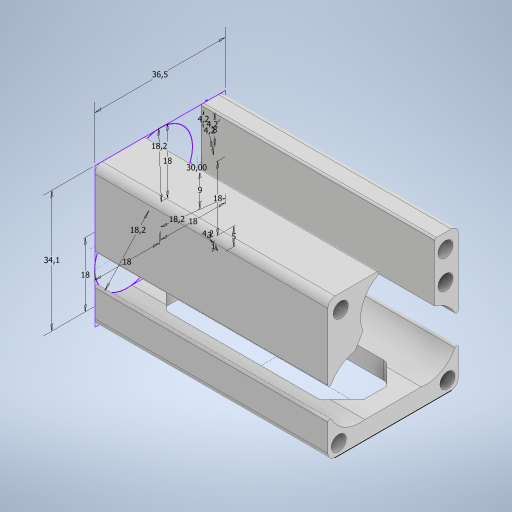
# Autodesk Inventor part: left_akkum
Saved by Autodesk Inventor 2023 (Build 270158000, 158)
## iProperties
Created: 2026-02-15
Part Number: left_akkum
Material: Типовые
Document SubType Name: Modeling
Designer: garin
Density: 1 g/cm^3
Appearance: По умолчанию
Author: garin
Autodesk Inventor part; units mm, degrees
ref_plane "YZ Plane" through (0, 0, 0) normal (1, 0, 0) x (0, 1, 0)
ref_plane "XZ Plane" through (0, 0, 0) normal (0, 1, 0) x (-1, 0, 0)
sketch "Эскиз1" plane through (0, 0, 0) normal (1, 0, 0) x (0, 1, 0)
  line L0 (-16.6, -18.25) -> (17.5, -18.25)
  line L1 (17.5, -18.25) -> (17.5, 18.25)
  line L2 (17.5, 18.25) -> (-16.6, 18.25)
  line L3 (-16.6, 18.25) -> (-16.6, -18.25)
  line L4 (17.5, 0) -> (-0.5, 0) construction
  circle A0 centre (8.5, 0) radius 9
  line L5 (-16.6, -18.25) -> (1.4, -18.25) construction
  line L6 (-7.6, -18.25) -> (-7.6, -0.25) construction
  circle A1 centre (-7.6, -9.25) radius 9
  line L7 (-16.6, 18.25) -> (1.4, 18.25) construction
  line L8 (-7.6, 18.25) -> (-7.6, 0.25) construction
  circle A2 centre (-7.6, 9.25) radius 9
  line L9 (-16.6, -18.25) -> (-16.6, -15.75)
  line L10 (-16.6, 18.25) -> (-21.6, 18.25)
  line L11 (-21.6, 18.25) -> (-21.6, -18.25)
  line L12 (-21.6, -18.25) -> (-16.6, -18.25)
  line L13 (-16.6, -18.25) -> (-16.6, 18.25)
  circle A3 centre (-18.6, -15.2) radius 1.5
  circle A4 centre (-18.6, -15.2) radius 2.1
  line L14 (-21.6, 18.25) -> (17.5, 18.25) construction
  line L15 (-2.05, 18.25) -> (-2.05, -18.25) construction
  circle A5 centre (13.4, -14.65) radius 1.5
  circle A6 centre (13.4, -14.65) radius 2.1
  circle A7 centre (8.5, 0) radius 9.1
  circle A8 centre (-7.6, 9.25) radius 9.1
  circle A9 centre (-7.6, -9.25) radius 9.1
  line L16 (-7.6, -0.15) -> (1.4, -0.15) construction
  line L17 (1.4, -0.15) -> (1.4, -10.5954) construction
  line L18 (1.4, -10.5954) -> (-7.6, -10.5954) construction
  line L19 (-7.6, -10.5954) -> (-7.6, -0.15) construction
  line L20 (1.4, -10.5954) -> (5.1186, -8.4484)
  line L21 (1.4, -10.5954) -> (5.6939, -10.5954) construction
  line L22 (1.4, 10.5954) -> (5.1186, 8.4484)
  line L23 (-16.7, 9.25) -> (-21.6, 9.25)
  line L24 (-16.7, -9.25) -> (-21.6, -9.25)
  line L25 (17.5, -11.65) -> (1.2036, -11.5536)
  line L26 (15.5, -18.25) -> (15.5, -11.6382) construction
  line L27 (11.3933, -16.75) -> (17.6, -16.75) construction
  line L28 (15.5, -16.75) -> (11.3, -16.75) construction
  line L29 (11.3, -16.75) -> (11.3, -12.55) construction
  line L30 (11.3, -12.55) -> (15.5, -12.55) construction
  line L31 (15.5, -12.55) -> (15.5, -16.75) construction
  line L32 (15.5, -14.65) -> (11.3, -14.65) construction
  line L33 (13.4, -12.55) -> (13.4, -16.75) construction
  circle A10 centre (13.4, 14.65) radius 1.5
  circle A11 centre (13.4, 14.65) radius 2.1
  line L34 (13.4, -14.65) -> (-21.6, -14.65) construction
  line L35 (-18.1, -14.65) -> (-19.1, -14.65) construction
  line L36 (-19.1, -15.75) -> (-18.1, -14.65) construction
  circle A12 centre (-18.6, 15.2) radius 1.5
  circle A13 centre (-18.6, 15.2) radius 2.1
  line L37 (13.4, -14.65) -> (5.4, -14.65)
  circle A14 centre (5.4, -14.65) radius 2.1
  point P0 (0, 0)
  point P1 (-8.9454, -18.25)
  point P2 (-8.9454, 18.25)
  point P3 (-6.2546, -18.25)
  point P4 (17.5, -1.3454)
  point P5 (17.5, 1.3454)
  point P6 (-6.2546, 18.25)
  point P7 (0.6455, -13.1)
  point P8 (17.5, -13.1)
  point P9 (-16.6, -7.9046)
  point P10 (-16.6, 7.9046)
  point P11 (-16.6, -10.5954)
  dimension "d13" = 18.2
  dimension "d14" = 18.2
  dimension "d0" = 34.1
  dimension "d1" = 36.5
  dimension "d2" = 18
  dimension "d3" = 18
  dimension "d4" = 18
  dimension "d5" = 18
  dimension "d6" = 18
  dimension "d8" = 5
  dimension "d11" = 3
  dimension "d12" = 4.2
  dimension "d15" = 18.2
  dimension "d16" = 9
  dimension "d17" = 30
  dimension "d27" = 4.2
  dimension "d28" = 4.2
  dimension "d29" = 1
  dimension "d48" = 8
  dimension "d49" = 4.2
  constraints: 76 end point, 18 point on line, 13 midpoint, 10 centre point, 9 coincident, 9 perpendicular, 8 parallel, 6 symmetric about line, 5 horizontal, 5 point on circle, 2 vertical alignment, 1 collinear, 1 equal length, 1 horizontal alignment, 1 vertical, 16 other
  measures "d0" distance of L2.end L1.end
  measures "d1" distance of L1.end L0.end
  measures "d2" distance of L4.start L4.end
  measures "d3" distance of L0.start L5.end
  measures "d4" distance of L6.start L6.end
  measures "d5" distance of L2.end L7.end
  measures "d6" distance of L8.start L8.end
  measures "d8" distance of L12.end L11.end
  measures "d11" diameter of A3
  measures "d12" diameter of A4
  measures "d15" diameter of A9
  measures "d16" distance of L17.end L18.end
  measures "d17" angle of L21 L20
  measures "d27" distance of L29.end L30.end
  measures "d28" distance of L28.end L29.end
  measures "d29" distance of L35.start L35.end
  measures "d48" distance of L34.start L37.end
  measures "d49" diameter of A14
extrude "Выдавливание3" add sketch "Эскиз1" along normal blind 65.2 contours L3 A4 A9 L0 | L12 L11 L24 A9 L3 A4 | A9 L25 L1 L0 | L11 L10 L3 A13 A8 L23 | L2 A8 L3 A13 | L22 A8 L2 L1 A7
extrude "Выдавливание4" add sketch "Эскиз1" along normal blind 5 contours L11 L23 A8 L3 A9 L24
extrude "Выдавливание5" add sketch "Эскиз1" against normal blind 5 from surface at 65.2 contours L11 L23 A8 L3 A9 L24
fillet "Сопряжение2" radius 2 4 edges at (32.6, 17.5, -18.25) (32.6, 17.5, 18.25) (32.6, -21.6, -18.25) (32.6, -21.6, 18.25)
ref_plane "РабПлоскость1" through (0, -21.6, 16.25) normal (0, -1, 0) x (1, 0, 0)
fillet "Сопряжение3" radius 0.5 6 edges at (32.6, 17.5, -11.65) (32.6, 17.5, 1.3454) (32.6, -6.2546, 18.25) (32.6, -8.9454, 18.25) (32.6, -6.2546, -18.25) (32.6, -8.9454, -18.25)
sketch "Эскиз2" plane through (0, -21.6, -16.25) normal (0, -1, 0) x (1, 0, 0)
  point P0 (0, 16.25)
chamfer "Фаска2" distance 6 angle 45 4 edges at (60.2, -19.15, -9.25) (60.2, -19.15, 9.25) (5, -19.15, -9.25) (5, -19.15, 9.25)
fillet "Сопряжение4" radius 2 4 edges at (54.2, -19.15, 9.25) (54.2, -19.15, -9.25) (11, -19.15, -9.25) (11, -19.15, 9.25)
sketch "Эскиз3" plane through (0, -21.6, 16.25) normal (0, -1, 0) x (1, 0, 0)
  point P0 (0, -16.25)
sketch "Эскиз4" plane through (0, -21.6, -16.25) normal (0, -1, 0) x (1, 0, 0)
  line L0 (65.2, 0) -> (0, 0) projected
  line L1 (0, 32.5) -> (65.2, 32.5) projected
  line L2 (0, 0) -> (65.2, 0)
  line L3 (65.2, 0) -> (65.2, 32.5)
  line L4 (65.2, 32.5) -> (0, 32.5)
  line L5 (0, 32.5) -> (0, 0)
  line L6 (65.2, 32.5) -> (65.2, 0) construction
  line L7 (65.2, 16.25) -> (0, 16.25) construction
  line L8 (32.6, 32.5) -> (32.6, 0) construction
  constraints: 12 end point, 3 midpoint, 2 horizontal, 2 parallel, 1 perpendicular
